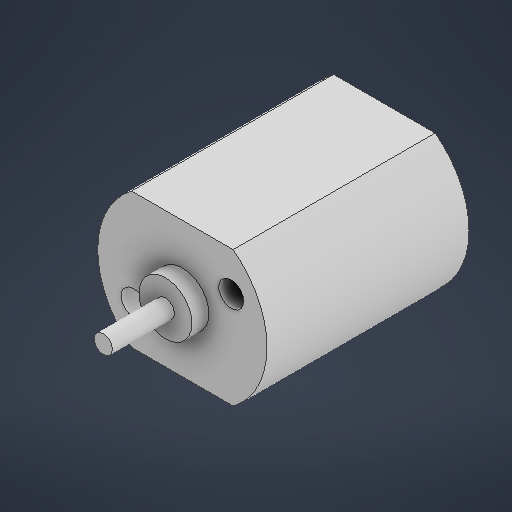
# Autodesk Inventor part: Silnik
Saved by Autodesk Inventor 2026 (Build 300175000, 175)
## iProperties
Created: 2025-04-26
Part Number: Silnik
Material: Generic
Document SubType Name: Modeling
Designer: isan
Density: 1 g/cm^3
Appearance: Default
Author: isan
Autodesk Inventor part; units mm, degrees
ref_plane "YZ Plane" through (0, 0, 0) normal (1, 0, 0) x (0, 1, 0)
ref_plane "XZ Plane" through (0, 0, 0) normal (0, 1, 0) x (-1, 0, 0)
ref_plane "XY Plane" through (0, 0, 0) normal (0, 0, 1) x (1, 0, 0)
sketch "Sketch1" plane through (0, 0, 0) normal (0, 1, 0) x (-1, 0, 0)
  circle A0 centre (0, 0) radius 7.5
  line L0 (10, -6) -> (-10, -6)
  line L1 (-10, -6) -> (-10, 6)
  line L2 (-10, 6) -> (10, 6)
  line L3 (10, 6) -> (10, -6)
  line L4 (10, -6) -> (-10, 6) construction
  line L5 (-10, -6) -> (10, 6) construction
  point P0 (4.5, 6)
  point P1 (-4.5, 6)
  point P2 (-4.5, -6)
  point P3 (4.5, -6)
  dimension "d0" = 15
  dimension "d1" = 12
  dimension "d2" = 20
  constraints: 12 end point, 2 midpoint, 2 parallel, 1 centre point, 1 coincident, 1 horizontal, 1 perpendicular
  measures "d0" diameter of A0
  measures "d1" distance of L0.end L1.end
  measures "d2" distance of L0.start L0.end
extrude "Extrusion1" add sketch "Sketch1" along normal blind 17.9 contours A0 L0 L2
sketch "Sketch2" plane through (0, 0, 0) normal (0, -1, 0) x (1, 0, 0)
  circle A0 centre (0, 0) radius 2.35
  dimension "d5" = 4.7
  constraints: 1 centre point, 1 coincident
  measures "d5" diameter of A0
extrude "Extrusion2" add sketch "Sketch2" along normal blind 1.5
sketch "Sketch3" plane through (0, -1.5, 0) normal (0, -1, 0) x (1, 0, 0)
  circle A0 centre (0, 0) radius 0.8
  dimension "d8" = 1.6
  constraints: 1 centre point, 1 coincident
  measures "d8" diameter of A0
extrude "Extrusion3" add sketch "Sketch3" along normal blind 5.5
sketch "Sketch4" plane through (0, 17.9, 0) normal (0, 1, 0) x (1, 0, 0)
  circle A0 centre (0, 0) radius 0.8 projected
  circle A1 centre (0, 0) radius 2.5
  dimension "d11" = 5
  constraints: 1 centre point, 1 coincident
  measures "d11" diameter of A1
extrude "Extrusion4" add sketch "Sketch4" along normal blind 0.7 contours A0 | A1
sketch "Sketch6" plane through (0, 17.9, 0) normal (0, 1, 0) x (1, 0, 0)
  line L0 (4.6211, -0.2655) -> (4.345, -0.3827)
  line L1 (4.345, -0.3827) -> (3.7589, 0.998)
  line L2 (3.7589, 0.998) -> (4.035, 1.1153)
  line L3 (4.035, 1.1153) -> (4.6211, -0.2655)
  line L4 (4.6211, -0.2655) -> (3.7589, 0.998) construction
  line L5 (4.345, -0.3827) -> (4.035, 1.1153) construction
  line L6 (-4.345, 0.3827) -> (-4.6211, 0.2655)
  line L7 (-4.6211, 0.2655) -> (-4.035, -1.1153)
  line L8 (-4.035, -1.1153) -> (-3.7589, -0.998)
  line L9 (-3.7589, -0.998) -> (-4.345, 0.3827)
  line L10 (-4.345, 0.3827) -> (-4.035, -1.1153) construction
  line L11 (-4.6211, 0.2655) -> (-3.7589, -0.998) construction
  point P0 (0, 0)
  point P1 (4.19, 0.3663)
  point P2 (-4.19, -0.3663)
  dimension "d26" = 0.3
  dimension "d27" = 1.5
  dimension "d28" = 0.3
  dimension "d29" = 1.5
  dimension "d30" = 4.19
  dimension "d31" = 4.19
  dimension "d32" = -0.3663
  dimension "d33" = -0.3663
  constraints: 24 end point, 4 midpoint, 4 parallel, 2 perpendicular
  measures "d26" distance of L0.start L0.end
  measures "d27" distance of L2.end L0.start
  measures "d28" distance of L7.end L8.end
  measures "d29" distance of L8.end L6.start
  measures "d30" horizontal distance of point (0, 0) point (-4.19, -0.366)
  measures "d31" horizontal distance of point (0, 0) point (4.19, 0.366)
  measures "d32" vertical distance of point (0, 0) point (4.19, 0.366)
  measures "d33" vertical distance of point (0, 0) point (-4.19, -0.366)
extrude "Extrusion5" add sketch "Sketch6" along normal blind 2.15
sketch "Sketch7" plane through (0, 0, 0) normal (0, -1, 0) x (1, 0, 0)
  line L0 (-6.7346, -3.8882) -> (6.7346, 3.8882) construction
  circle A0 centre (-4.3301, -2.5) radius 1.1
  circle A1 centre (4.3301, 2.5) radius 1.1
  point P0 (0, 0)
  point P1 (0, 0)
  dimension "d36" = 2.2
  dimension "d37" = 2.2
  dimension "d38" = 5
  dimension "d39" = 5
  constraints: 2 centre point, 2 end point, 2 point on line, 1 midpoint
  measures "d36" diameter of A0
  measures "d37" diameter of A1
  measures "d38" distance of point (0, 0) A0.centre
  measures "d39" distance of point (0, 0) A1.centre
extrude "Extrusion6" cut sketch "Sketch7" against normal blind 2.15
body "Solid1"
